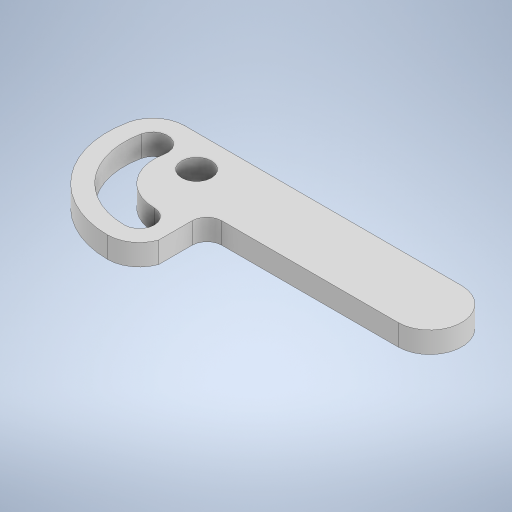
# Autodesk Inventor part: Assignment#1
Saved by Autodesk Inventor 2023.2 (Build 272271000, 271)
## iProperties
Created: 2023-01-17
Part Number: Assignment#1
Material: Generic
Document SubType Name: Modeling
Designer: manas
Density: 1 g/cm^3
Appearance: Default
Author: manas
Autodesk Inventor part; units mm, degrees
ref_plane "YZ Plane" through (0, 0, 0) normal (1, 0, 0) x (0, 1, 0)
ref_plane "XZ Plane" through (0, 0, 0) normal (0, 1, 0) x (-1, 0, 0)
ref_plane "XY Plane" through (0, 0, 0) normal (0, 0, 1) x (1, 0, 0)
sketch "Sketch1" plane through (0, 0, 0) normal (0, 1, 0) x (-1, 0, 0)
  arc A0 (0, 15) -> (0, -15) centre (0, 0) ccw
  line L0 (0, -15) -> (130.51, -15)
  line L1 (0, 15) -> (83, 15)
  arc A1 (130.51, -15) -> (145.1737, -3.1586) centre (130.51, 0) ccw
  arc A2 (123.667, 1.474) -> (137.353, -1.474) centre (130.51, 0) ccw
  circle A3 centre (109.88, 0) radius 7
  arc A4 (123.667, 1.474) -> (104.1154, 25.6855) centre (104.1154, 5.6855) ccw
  arc A5 (104.1154, 39.6855) -> (104.1154, 25.6855) centre (104.1154, 32.6855) ccw
  arc A6 (137.353, -1.474) -> (104.1154, 39.6855) centre (104.1154, 5.6855) ccw
  arc A7 (104.1154, 47.6855) -> (90, 37.7605) centre (104.1154, 32.6855) ccw
  line L2 (90, 22) -> (90, 37.7605)
  arc A8 (145.1737, -3.1586) -> (104.1154, 47.6855) centre (104.1154, 5.6855) ccw
  arc A9 (83, 15) -> (90, 22) centre (83, 22) ccw
  point P0 (90, 15)
  dimension "d0" = 30
  dimension "d1" = 130.51
  dimension "d2" = 90
  dimension "d3" = 15
  dimension "d4" = 14
  dimension "d5" = 20.63
  dimension "d6" = 14
  dimension "d9" = 20
  dimension "d11" = 14
  dimension "d12" = 15
  dimension "d13" = 42
  dimension "d14" = 7
  constraints: 18 point on circle, 10 centre point, 10 tangent, 6 end point, 4 coincident, 2 horizontal, 2 point on line, 1 vertical
  measures "d0" diameter of A0
  measures "d1" distance of L0.start L0.end
  measures "d2" distance of L1.start point (90, 15)
  measures "d3" radius of A1
  measures "d4" diameter of A2
  measures "d5" distance of A3.centre A1.centre
  measures "d6" diameter of A3
  measures "d9" radius of A4
  measures "d11" diameter of A5
  measures "d12" radius of A7
  measures "d13" radius of A8
  measures "d14" radius of A9
extrude "Extrusion1" add sketch "Sketch1" along normal blind 10
body "Solid1"
